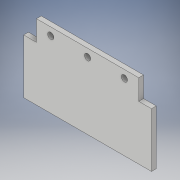
# Autodesk Inventor part: Top
Saved by Autodesk Inventor 2018 (Build 220112000, 112)
## iProperties
Created: 2018-04-18
Part Number: Top
Material: Generic
Document SubType Name: Modeling
Designer: trent
Density: 1 g/cm^3
Appearance: Default
Author: trent
Autodesk Inventor part; units mm, degrees
ref_plane "YZ Plane" through (0, 0, 0) normal (1, 0, 0) x (0, 1, 0)
ref_plane "XZ Plane" through (0, 0, 0) normal (0, 1, 0) x (-1, 0, 0)
ref_plane "XY Plane" through (0, 0, 0) normal (0, 0, 1) x (1, 0, 0)
sketch "Sketch1" plane through (0, 0, 0) normal (0, 0, 1) x (1, 0, 0)
  line L0 (0, 0) -> (127, 0)
  line L1 (127, 0) -> (127, 53.975)
  line L2 (127, 53.975) -> (0, 53.975)
  line L3 (0, 53.975) -> (0, 0)
  line L4 (12.7, 53.975) -> (114.3, 53.975)
  line L5 (114.3, 53.975) -> (114.3, 74.295)
  line L6 (114.3, 74.295) -> (12.7, 74.295)
  line L7 (12.7, 74.295) -> (12.7, 53.975)
  circle A0 centre (26.924, 66.675) radius 3.0988
  circle A1 centre (63.5, 66.675) radius 3.0988
  circle A2 centre (100.076, 66.675) radius 3.0988
  dimension "d0" = 127
  dimension "d1" = 53.975
  dimension "d2" = 101.6
  dimension "d3" = 12.7
  dimension "d4" = 20.32
  dimension "d5" = 6.1976
  dimension "d6" = 36.576
  dimension "d12" = 12.7
  dimension "d13" = 12.7
  dimension "d14" = 50.8
  dimension "d15" = 12.7
  dimension "d16" = 36.576
  constraints: 16 end point, 4 parallel, 3 centre point, 2 equal radius, 2 horizontal, 2 perpendicular, 1 point on line
  measures "d0" distance of L2.end L1.end
  measures "d1" distance of L1.end L0.end
  measures "d2" distance of L6.end L5.end
  measures "d3" distance between parallel lines of L3 L7
  measures "d4" distance between parallel lines of L2 L6
  measures "d5" diameter of A0
  measures "d6" distance of A1.centre A0.centre
  measures "d12" distance from line of L2 A0.centre
  measures "d13" distance from line of L2 A1.centre
  measures "d14" distance from line of L7 A1.centre
  measures "d15" distance from line of L2 A2.centre
  measures "d16" distance of A1.centre A2.centre
extrude "Extrusion1" add sketch "Sketch1" along normal blind 4.7625
equation "\"d3\" = -0.5 * d2 + 0.5 * d0"
equation "\"d13\" = d12"
equation "\"d14\" = 0.5 * d2"
equation "\"d15\" = d13"
equation "\"d16\" = d6"
body "Solid1"
